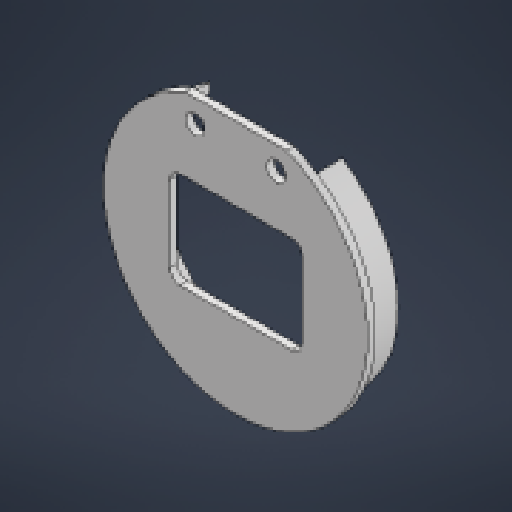
# Autodesk Inventor part: Mirror_Mount
Saved by Autodesk Inventor 2024.2 (Build 282272000, 272)
## iProperties
Created: 2023-12-21
Part Number: Mirror_Mount
Material: 一般
Document SubType Name: Modeling
Designer: Hanaoka
Density: 1 g/cm^3
Appearance: 既定
Author: Hanaoka
Autodesk Inventor part; units mm, degrees
ref_plane "YZ Plane" through (0, 0, 0) normal (1, 0, 0) x (0, 1, 0)
ref_plane "作業平面1" through (0, 0, 0) normal (0, 0, 1) x (1, 0, 0)
ref_plane "作業平面2" through (0, 0, -8.3) normal (0, 0, -1) x (-1, 0, 0)
sketch "スケッチ1" plane through (0, 0, -8.3) normal (0, 0, -1) x (-1, 0, 0)
  circle A0 centre (0, -11.25) radius 6.5 projected
  circle A1 centre (0, -11.25) radius 26
  line L0 (10, 12.75) -> (-10, 12.75)
  line L1 (11, -1.75) -> (-11, -1.75)
  line L2 (-13, -3.75) -> (-13, -18.75)
  line L3 (-11, -20.75) -> (11, -20.75)
  line L4 (13, -18.75) -> (13, -3.75)
  line L5 (13, -1.75) -> (-13, -20.75) construction
  line L6 (-13, -1.75) -> (13, -20.75) construction
  arc A2 (11, -20.75) -> (13, -18.75) centre (11, -18.75) ccw
  arc A3 (13, -3.75) -> (11, -1.75) centre (11, -3.75) ccw
  arc A4 (-11, -1.75) -> (-13, -3.75) centre (-11, -3.75) ccw
  arc A5 (-13, -18.75) -> (-11, -20.75) centre (-11, -18.75) ccw
  circle A6 centre (8, 8.2) radius 2.425 projected
  circle A7 centre (-8, 8.2) radius 2.425 projected
  circle A8 centre (8, 8.2) radius 1.875
  circle A9 centre (-8, 8.2) radius 1.875
  point P0 (0, 0)
  dimension "d0" = 52
  dimension "d1" = 20
  dimension "d2" = 26
  dimension "d3" = 19
  dimension "d4" = 2
  dimension "d7" = 3.75
  constraints: 14 end point, 10 point on circle, 8 point on line, 8 tangent, 7 centre point, 4 equal radius, 3 coincident, 2 horizontal, 2 midpoint, 2 parallel, 1 perpendicular
  measures "d0" diameter of A1
  measures "d1" distance of L0.start L0.end
  measures "d2" distance of L5.end L6.end
  measures "d3" distance of L6.start L5.end
  measures "d4" radius of A2
  measures "d7" diameter of A8
extrude "押し出し1" add sketch "スケッチ1" along normal blind 1.5 contours A1 L0 | A6 | A7 picked at (-0.9365, -26.1993)
sketch "スケッチ2" plane through (0, 0, -8.3) normal (0, 0, 1) x (1, 0, 0)
  circle A0 centre (0, -11.25) radius 24
  arc A1 (-10, 12.75) -> (10, 12.75) centre (0, -11.25) ccw projected
  arc A2 (-13, 7.1144) -> (13, 7.1144) centre (0, -11.25) ccw
  line L0 (-13, 7.1144) -> (-13, 8.9242)
  line L1 (13, 7.1144) -> (13, 8.9242)
  point P0 (0, 0)
  point P1 (13, 8.0193)
  dimension "d8" = 48
  dimension "d9" = 1.5
  dimension "d10" = 26
  constraints: 4 end point, 4 point on circle, 2 centre point, 2 coincident, 2 parallel, 1 midpoint, 1 vertical
  measures "d8" diameter of A0
  measures "d9" radial gap between concentric circles of A2 A0
  measures "d10" distance from line of point (13, 8.019) L0
extrude "押し出し2" add sketch "スケッチ2" against normal blind 8 contours A0 L0 A2 L1 picked at (18.6222, -25.3282)
